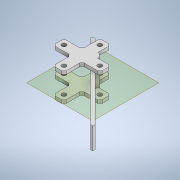
# Autodesk Inventor part: Holder
Saved by Autodesk Inventor 2020 (Build 240168000, 168)
## iProperties
Created: 2019-12-20
Part Number: Holder
Material: Generic
Document SubType Name: Modeling
Designer: atmat
Density: 1 g/cm^3
Appearance: Default
Author: atmat
Autodesk Inventor part; units mm, degrees
ref_plane "YZ Plane" through (0, 0, 0) normal (1, 0, 0) x (0, 1, 0)
ref_plane "XZ Plane" through (0, 0, 0) normal (0, 1, 0) x (-1, 0, 0)
ref_plane "XY Plane" through (0, 0, 0) normal (0, 0, 1) x (1, 0, 0)
sketch "Sketch1" plane through (0, 0, 0) normal (0, 1, 0) x (-1, 0, 0)
  circle A0 centre (0, 16.5) radius 2
  circle A1 centre (0, -16.5) radius 2
  circle A2 centre (16.5, 0) radius 2
  circle A3 centre (-16.5, 0) radius 2
  line L0 (5, 21.5) -> (-5, 21.5)
  line L1 (-5, 21.5) -> (-5, -21.5)
  line L2 (-5, -21.5) -> (5, -21.5)
  line L3 (5, -21.5) -> (5, 21.5)
  line L4 (21.5, 5) -> (-21.5, 5)
  line L5 (-21.5, 5) -> (-21.5, -5)
  line L6 (-21.5, -5) -> (21.5, -5)
  line L7 (21.5, -5) -> (21.5, 5)
  point P0 (0, 0)
  point P1 (-5, 5)
  point P2 (-5, -5)
  point P3 (5, -5)
  point P4 (5, 5)
  dimension "d0" = 4
  dimension "d1" = 4
  dimension "d2" = 16.5
  dimension "d3" = 16.5
  dimension "d4" = 4
  dimension "d5" = 4
  dimension "d6" = 16.5
  dimension "d7" = 16.5
  dimension "d8" = 3
  dimension "d9" = 10
  dimension "d10" = 3
  dimension "d11" = 3
  dimension "d12" = 5
  dimension "d13" = 5
  dimension "d14" = 5
  dimension "d15" = 5
  constraints: 16 end point, 4 centre point, 4 parallel, 2 horizontal, 2 perpendicular
  measures "d0" diameter of A0
  measures "d1" diameter of A1
  measures "d2" distance of point (0, 0) A0.centre
  measures "d3" distance of point (0, 0) A1.centre
  measures "d4" diameter of A2
  measures "d5" diameter of A3
  measures "d6" distance of point (0, 0) A2.centre
  measures "d7" distance of point (0, 0) A3.centre
  measures "d8" distance edge to line of A0 L3
  measures "d9" distance between parallel lines of L3 L1
  measures "d10" distance edge to line of A0 L0
  measures "d11" distance edge to line of A1 L2
  measures "d12" distance from line of L4 A2.centre
  measures "d13" distance from line of A2.centre L6
  measures "d14" distance from line of A2.centre L7
  measures "d15" distance from line of A3.centre L5
extrude "Extrusion1" add sketch "Sketch1" along normal blind 3
chamfer "Chamfer1" distance 2 angle 45 12 edges at (5, 1.5, -21.5) (21.5, 1.5, -5) (21.5, 1.5, 5) (-5, 1.5, -21.5) (5, 1.5, -5) (-5, 1.5, -5) (-21.5, 1.5, -5) (-21.5, 1.5, 5) (-5, 1.5, 21.5) (-5, 1.5, 5) (5, 1.5, 21.5) (5, 1.5, 5)
sketch "Sketch3" plane through (0, 0, 0) normal (0, -1, 0) x (1, 0, 0)
  line L0 (-11.6777, -23.6777) -> (59.033, 47.033)
  line L1 (59.033, 47.033) -> (56.9117, 49.1543)
  line L2 (56.9117, 49.1543) -> (-13.799, -21.5563)
  line L3 (-7, 5) -> (-5, 7) projected
  line L4 (7, -5) -> (5, -7) projected
  line L5 (5, 7) -> (7, 5) projected
  line L6 (-5, -7) -> (-7, -5) projected
  line L7 (-11.6777, -23.6777) -> (-13.799, -21.5563)
  point P0 (0, 0)
  dimension "d25" = 0
  dimension "d26" = 3
  dimension "d27" = 25
  dimension "d28" = 75
  constraints: 8 end point, 3 parallel, 1 collinear
  measures "d25" distance between parallel lines of L4 L0
  measures "d26" distance between parallel lines of L0 L2
  measures "d27" distance from line of L7 point (0, 0)
  measures "d28" distance from line of point (0, 0) L1
extrude "Extrusion2" add sketch "Sketch3" along normal blind 10
ref_plane "Work Plane1" through (0, -10, 0) normal (0, -1, 0) x (1, 0, 0)
mirror "Mirror1" about plane through (0, -10, 0) normal (0, -1, 0) of "Extrusion1", "Chamfer1", "Extrusion2"
chamfer "Chamfer2" distance 1.5 angle 45 4 edges at (59.033, -10, 47.033) (56.9117, -10, 49.1543) (-11.6777, -10, -23.6777) (-13.799, -10, -21.5563)
sketch "Sketch4" plane through (5, 0, -7) normal (0.7071068, 0, -0.7071068) x (-0.7071068, 0, -0.7071068)
  line L0 (-11.6673, 3) -> (-2.8284, 3) projected
  line L1 (8.8388, -23) -> (0, -23) projected
  line L2 (-6.4142, 3) -> (3.5858, 3)
  line L3 (3.5858, 3) -> (3.5858, -23)
  line L4 (3.5858, -23) -> (-6.4142, -23)
  line L5 (-6.4142, -23) -> (-6.4142, 3)
  point P0 (-1.4142, 0)
  point P1 (0, -23)
  point P2 (-2.8284, 3)
  dimension "d35" = 5
  dimension "d36" = 5
  constraints: 8 end point, 2 parallel, 2 point on line, 1 horizontal, 1 perpendicular
  measures "d35" distance from line of point (-1.414, 0) L5
  measures "d36" distance from line of L3 point (-1.414, 0)
extrude "Extrusion3" add sketch "Sketch4" along normal blind 3
chamfer "Chamfer3" distance 3 angle 45 2 edges at (4.5858, -10, -11.6569) (11.6569, -10, -4.5858)
body "Solid1"
